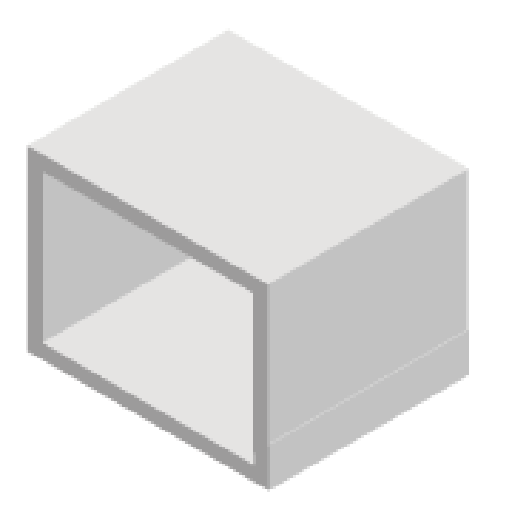
# Autodesk Inventor part: OpenFrameAdapter
Saved by Autodesk Inventor 2024.1 (Build 281209000, 209)
## iProperties
Created: 2021-06-08
Part Number: OpenFrameAdapter
Material: Generic
Document SubType Name: Modeling
Designer: wanghaoran
Density: 1 g/cm^3
Appearance: Default
Author: wanghaoran
Autodesk Inventor part; units mm, degrees
ref_plane "YZ Plane" through (0, 0, 0) normal (1, 0, 0) x (0, 1, 0)
ref_plane "XZ Plane" through (0, 0, 0) normal (0, 1, 0) x (-1, 0, 0)
ref_plane "XY Plane" through (0, 0, 0) normal (0, 0, 1) x (1, 0, 0)
ref_plane "Arbeitsebene3" through (60, 0, -82.935) normal (0, 0, 1) x (1, 0, 0)
sketch "Skizze13" plane through (60, 0, -82.935) normal (0, 0, 1) x (1, 0, 0)
  line L0 (-37.4166, 8.45) -> (-37.4166, 59.55) projected
  ellipse E0 centre (23.8014, -114.2521) end of major axis (147.0034, -54.0467) minor radius 137.1256 (-36.404, 8.95) -> (-37.4166, 8.45) ccw projected
  line L1 (-36.404, 8.95) -> (36.404, 8.95) projected
  ellipse E1 centre (-23.8014, -114.2521) end of major axis (98.9007, -175.47) minor radius 137.1256 (37.4166, 8.45) -> (36.404, 8.95) ccw projected
  line L2 (37.4166, 59.55) -> (37.4166, 8.45) projected
  ellipse E2 centre (-23.8014, 182.2521) end of major axis (-147.0034, 122.0467) minor radius 137.1256 (36.404, 59.05) -> (37.4166, 59.55) ccw projected
  line L3 (36.404, 59.05) -> (-36.404, 59.05) projected
  ellipse E3 centre (23.8014, 182.2521) end of major axis (-98.9007, 243.47) minor radius 137.1256 (-37.4166, 59.55) -> (-36.404, 59.05) ccw projected
  arc A0 (11.7926, 47.5991) -> (-11.7926, 47.5991) centre (0, 34) ccw projected
  arc A1 (13.5991, 45.7926) -> (11.7926, 47.5991) centre (15, 49) ccw projected
  arc A2 (13.5991, 22.2074) -> (13.5991, 45.7926) centre (0, 34) ccw projected
  arc A3 (11.7926, 20.4009) -> (13.5991, 22.2074) centre (15, 19) ccw projected
  arc A4 (-11.7926, 20.4009) -> (11.7926, 20.4009) centre (0, 34) ccw projected
  arc A5 (-13.5991, 22.2074) -> (-11.7926, 20.4009) centre (-15, 19) ccw projected
  arc A6 (-13.5991, 45.7926) -> (-13.5991, 22.2074) centre (0, 34) ccw projected
  arc A7 (-11.7926, 47.5991) -> (-13.5991, 45.7926) centre (-15, 49) ccw projected
  circle A8 centre (19, 15) radius 1.621 projected
  circle A9 centre (19, 53) radius 1.621 projected
  circle A10 centre (-19, 15) radius 1.621 projected
  circle A11 centre (-19, 53) radius 1.621 projected
  circle A12 centre (0, 34) radius 16
  line L4 (-33.4166, 58.05) -> (33.4166, 58.05)
  line L5 (36.4166, 55.05) -> (36.4166, 12.95)
  line L6 (33.4166, 9.95) -> (-33.4166, 9.95)
  line L7 (-36.4166, 12.95) -> (-36.4166, 55.05)
  arc A13 (-33.4166, 58.05) -> (-36.4166, 55.05) centre (-33.4166, 55.05) ccw
  arc A14 (-36.4166, 12.95) -> (-33.4166, 9.95) centre (-33.4166, 12.95) ccw
  arc A15 (33.4166, 9.95) -> (36.4166, 12.95) centre (33.4166, 12.95) ccw
  arc A16 (36.4166, 55.05) -> (33.4166, 58.05) centre (33.4166, 55.05) ccw
  point P0 (-60, 0)
  dimension "d147" = 32
  dimension "d148" = 1
  dimension "d149" = 3
  constraints: 8 end point, 8 point on circle, 8 tangent, 5 centre point, 3 equal radius, 1 coincident, 7 other
  measures "d147" diameter of A12
  measures "d148" distance between parallel lines of L3 L4
  measures "d149" radius of A13
extrude "Extrusion11" add sketch "Skizze13" along normal blind 8 contours A1 A2 A3 A4 A5 A6 A7 A0 | L4 A16 L5 A15 L6 A14 L7 A13
sketch "Skizze14" plane through (60, 0, -74.935) normal (0, 0, 1) x (1, 0, 0)
  point P0 (-60, 0)
sketch "Skizze15" plane through (60, 0, -74.935) normal (0, 0, 1) x (1, 0, 0)
  line L0 (-33.541, 7.75) -> (-33.541, 50.25)
  line L1 (-33.4166, 9.95) -> (33.4166, 9.95)
  arc A0 (33.4166, 9.95) -> (36.4166, 12.95) centre (33.4166, 12.95) ccw
  line L2 (36.4166, 12.95) -> (36.4166, 55.05)
  arc A1 (36.4166, 55.05) -> (33.4166, 58.05) centre (33.4166, 55.05) ccw
  line L3 (33.4166, 58.05) -> (-33.4166, 58.05)
  arc A2 (-33.4166, 58.05) -> (-36.4166, 55.05) centre (-33.4166, 55.05) ccw
  line L4 (-36.4166, 55.05) -> (-36.4166, 12.95)
  arc A3 (-36.4166, 12.95) -> (-33.4166, 9.95) centre (-33.4166, 12.95) ccw
  circle A4 centre (0, 34) radius 16
  circle A5 centre (-19, 53) radius 1.621
  circle A6 centre (-19, 15) radius 1.621
  circle A7 centre (19, 53) radius 1.621
  circle A8 centre (19, 15) radius 1.621
  line L5 (-77.5, 76.5) -> (77.5, 76.5)
  line L6 (-66, 79) -> (-60, 79)
  line L7 (66, -21) -> (66, 79)
  line L8 (-66, 79) -> (-66, -21)
  line L9 (-77.5, 107.3475) -> (77.5, 107.3475)
  line L10 (-33.4166, 9.95) -> (33.4166, 9.95)
  arc A9 (33.4166, 9.95) -> (36.4166, 12.95) centre (33.4166, 12.95) ccw
  line L11 (36.4166, 12.95) -> (36.4166, 55.05)
  arc A10 (36.4166, 55.05) -> (33.4166, 58.05) centre (33.4166, 55.05) ccw
  line L12 (33.4166, 58.05) -> (-33.4166, 58.05)
  arc A11 (-33.4166, 58.05) -> (-36.4166, 55.05) centre (-33.4166, 55.05) ccw
  line L13 (-36.4166, 55.05) -> (-36.4166, 12.95)
  arc A12 (-36.4166, 12.95) -> (-33.4166, 9.95) centre (-33.4166, 12.95) ccw
  circle A13 centre (0, 34) radius 16
  circle A14 centre (-19, 53) radius 1.621
  circle A15 centre (-19, 15) radius 1.621
  circle A16 centre (19, 53) radius 1.621
  circle A17 centre (19, 15) radius 1.621
  line L14 (-33.4166, 55.05) -> (33.4166, 55.05)
  line L15 (33.4166, 55.05) -> (33.4166, 12.95)
  line L16 (33.4166, 12.95) -> (-33.4166, 12.95)
  line L17 (-33.4166, 12.95) -> (-33.4166, 55.05)
  line L18 (60, -8) -> (-60, -8)
  line L19 (-60, -8) -> (-60, 76)
  line L20 (-60, 76) -> (60, 76)
  line L21 (60, 76) -> (60, -8)
  line L22 (60, -8) -> (-60, 76) construction
  line L23 (-60, -8) -> (60, 76) construction
  line L24 (-60, -8) -> (60, -8)
  line L25 (60, -8) -> (60, -21)
  line L26 (60, -21) -> (-60, -21)
  line L27 (-60, -21) -> (-60, -8)
  point P0 (-60, 0)
  point P1 (60, -8)
extrude "Extrusion12" add sketch "Skizze15" along normal blind 8 contours A3 L4 A2 L3 A1 L2 A0 L1 | L25 L26 L27 L18 | L18 L19 L20 L21
chamfer "Fasen1" distance 3 angle 45 4 edges at (93.4166, 34, -74.935) (60, 12.95, -74.935) (26.5834, 34, -74.935) (60, 55.05, -74.935)
sketch "Skizze16" plane through (60, 0, -66.935) normal (0, 0, 1) x (1, 0, 0)
  line L0 (60, 76) -> (-60, 76) projected
  line L1 (-60, 76) -> (-60, -21) projected
  line L2 (-60, -21) -> (60, -21) projected
  line L3 (60, -21) -> (60, 76) projected
  line L4 (-33.4166, 55.05) -> (33.4166, 55.05) projected
  line L5 (33.4166, 55.05) -> (33.4166, 12.95) projected
  line L6 (33.4166, 12.95) -> (-33.4166, 12.95) projected
  line L7 (-33.4166, 12.95) -> (-33.4166, 55.05) projected
  line L8 (-54, 70) -> (54, 70)
  line L9 (54, 70) -> (54, -15)
  line L10 (54, -15) -> (-54, -15)
  line L11 (-54, -15) -> (-54, 70)
  dimension "d163" = 6
  constraints: 8 end point, 3 other
  measures "d163" distance between parallel lines of L0 L8
extrude "Extrusion13" add sketch "Skizze16" along normal up to surface (101.4112 mm away) contours L3 L2 L1 L0
